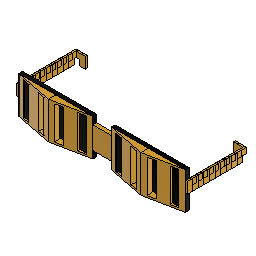
aizawaglasses v3 (Autodesk Fusion 360 design; units mm, degrees)
Autodesk Fusion 360 part; units mm, degrees
sketch "Sketch1" plane through (0, 0, 0) normal (0, 1, 0) x (1, 0, 0) in component "black"
  line L0 (0, 0) -> (50.8, 0)
  line L1 (50.8, 0) -> (50.8, -25.4)
  line L2 (50.8, -25.4) -> (0, -25.4)
  line L3 (0, -25.4) -> (0, 0)
  dimension "d1" = 50.8
  dimension "d2" = 25.4
  constraint horizontal L0
  constraint vertical L1
  constraint horizontal L2
  constraint vertical L3
  constraint coincident L0.start L3.end
  measures "d1" distance of L1.end L2.end
  measures "d2" distance of L0.start L2.end
extrude "Extrude1" add sketch "Sketch1" along normal blind 2.54 makes body 1 in component "black"
sketch "Sketch1 (2)" plane through (0, 0, 0) normal (0, 0, -1) x (1, 0, 0) in component "goggle"
  line L0 (50.8, 0) -> (0, 0)
  line L1 (0, 0) -> (0, -2.54)
  line L2 (0, -2.54) -> (50.8, -2.54)
  line L3 (50.8, -2.54) -> (50.8, 0)
  line L4 (25.4, 0) -> (25.4, 5.08)
  line L5 (25.4, 5.08) -> (50.8, 0)
  dimension "d5" = 5.08
  constraint midpoint L0 L4.start
  constraint perpendicular L0 L4
  constraint coincident L0.start L3.end
  measures "d5" distance of L4.start L4.end
extrude "Extrude1'" add sketch "Sketch1 (2)" against normal blind 25.4 separate body contours L0 L4 L5 makes body 2 in component "goggle"
copy_body "CopyPasteBodies1" bodies 2 makes body 3 in component "goggle"
move_body "Move1" bodies 3 to x (-1, 0, 0) y (0, 1, 0) z (0, 0, -1) at (50.8, 0, 27.056) in component "goggle"
move_body "Move2" bodies 3 to x (1, 0, 0) y (0, 1, 0) z (0, 0, 1) at (0, 0, -1.656) in component "goggle"
sketch "Sketch2" plane through (0, 0, 0) normal (-0.196116, -0.980581, 0) x (0.980581, -0.196116, 0) in component "goggle"
  line L0 (25.903, 25.4) -> (0, 25.4)
  line L1 (0, 25.4) -> (0, 0)
  line L2 (0, 0) -> (25.903, 0)
  line L3 (25.903, 0) -> (25.903, 25.4)
  line L4 (3.81, 24.13) -> (8.89, 24.13)
  line L5 (8.89, 24.13) -> (8.89, 1.27)
  line L6 (8.89, 1.27) -> (3.81, 1.27)
  line L7 (3.81, 1.27) -> (3.81, 24.13)
  line L8 (17.013, 24.13) -> (22.093, 24.13)
  line L9 (22.093, 24.13) -> (22.093, 1.27)
  line L10 (22.093, 1.27) -> (17.013, 1.27)
  line L11 (17.013, 1.27) -> (17.013, 24.13)
  dimension "d8" = 22.86
  dimension "d9" = 5.08
  dimension "d10" = 22.86
  dimension "d11" = 5.08
  dimension "d12" = 3.81
  dimension "d13" = 3.81
  dimension "d14" = 1.27
  dimension "d15" = 1.27
  constraint horizontal L4
  constraint vertical L5
  constraint horizontal L6
  constraint vertical L7
  constraint horizontal L8
  constraint vertical L9
  constraint horizontal L10
  constraint vertical L11
  measures "d8" distance of L8.start L10.end
  measures "d9" distance of L8.start L8.end
  measures "d10" distance of L4.start L6.end
  measures "d11" distance of L4.start L4.end
  measures "d12" distance of L1 L7
  measures "d13" distance of L3 L9
  measures "d14" distance of L0 L4
  measures "d15" distance of L0 L8
extrude "Extrude2" cut sketch "Sketch2" against normal blind 7.62 contours L4 L5 L6 L7 | L8 L9 L10 L11 bodies 3 in component "goggle"
sketch "Sketch3" plane through (1.9538, -9.7692, 0) normal (0.196116, -0.980581, 0) x (0.980581, 0.196116, 0) in component "goggle"
  line L0 (23.9105, 0) -> (49.8135, 0)
  line L1 (49.8135, 0) -> (49.8135, 25.4)
  line L2 (49.8135, 25.4) -> (23.9105, 25.4)
  line L3 (23.9105, 25.4) -> (23.9105, 0)
  line L4 (27.7205, 24.13) -> (32.8005, 24.13)
  line L5 (32.8005, 24.13) -> (32.8005, 1.27)
  line L6 (32.8005, 1.27) -> (27.7205, 1.27)
  line L7 (27.7205, 1.27) -> (27.7205, 24.13)
  line L8 (40.9235, 24.13) -> (46.0035, 24.13)
  line L9 (46.0035, 24.13) -> (46.0035, 1.27)
  line L10 (46.0035, 1.27) -> (40.9235, 1.27)
  line L11 (40.9235, 1.27) -> (40.9235, 24.13)
  dimension "d18" = 22.86
  dimension "d19" = 5.08
  dimension "d20" = 3.81
  dimension "d21" = 1.27
  dimension "d22" = 22.86
  dimension "d23" = 5.08
  dimension "d24" = 1.27
  dimension "d25" = 3.81
  constraint horizontal L4
  constraint vertical L5
  constraint horizontal L6
  constraint vertical L7
  constraint horizontal L8
  constraint vertical L9
  constraint horizontal L10
  constraint vertical L11
  measures "d18" distance of L4.start L6.end
  measures "d19" distance of L4.start L4.end
  measures "d20" distance of L3 L7
  measures "d21" distance of L2 L4
  measures "d22" distance of L8.start L10.end
  measures "d23" distance of L8.start L8.end
  measures "d24" distance of L2 L8
  measures "d25" distance of L1 L9
extrude "Extrude3" cut sketch "Sketch3" against normal blind 10.16 contours L4 L5 L6 L7 | L8 L9 L10 L11 bodies 2 in component "goggle"
sketch "Sketch1 (3)" plane through (50.8, 0, 0) normal (1, 0, 0) x (0, 1, 0)
  line L0 (0, 25.4) -> (0, 0)
  line L1 (0, 0) -> (2.54, 0)
  line L2 (2.54, 0) -> (2.54, 25.4)
  line L3 (2.54, 25.4) -> (0, 25.4)
  line L4 (0, 20.32) -> (2.54, 20.32)
  line L5 (2.54, 20.32) -> (2.54, 5.08)
  line L6 (2.54, 5.08) -> (0, 5.08)
  line L7 (0, 5.08) -> (0, 20.32)
  constraint horizontal L4
  constraint vertical L5
  constraint horizontal L6
  constraint vertical L7
  constraint coincident L2 L5.end
  constraint coincident L0 L4.start
extrude "Extrude1''" add sketch "Sketch1 (3)" along normal blind 12.7 separate body contours L0 L2 L4 L5 L6 L7 makes body 4
copy_body "CutPasteBodies1" bodies 4 removing the originals makes body 5 in component "strap"
copy_body "CopyPasteBodies1'" bodies 2 1 3 makes body 6 makes body 7 makes body 8
move_body "Move1'" bodies 6 7 8 to x (1, 0, 0) y (0, 1, 0) z (0, 0, 1) at (63.5, 0, 0)
sketch "Sketch2 (2)" plane through (114.3, 0, 0) normal (1, 0, 0) x (0, 1, 0) in component "strap"
  line L0 (0, 25.4) -> (0, 0)
  line L1 (0, 0) -> (2.54, 0)
  line L2 (2.54, 0) -> (2.54, 25.4)
  line L3 (2.54, 25.4) -> (0, 25.4)
  line L4 (0, 19.1041) -> (52.113, 19.1041)
  line L5 (52.113, 19.1041) -> (52.113, 11.4841)
  line L6 (52.113, 11.4841) -> (0, 11.4841)
  line L7 (0, 11.4841) -> (0, 19.1041)
  dimension "d30" = 7.62
  constraint horizontal L4
  constraint vertical L5
  constraint horizontal L6
  constraint vertical L7
  constraint coincident L0 L4.start
  measures "d30" distance of L4.start L6.end
sketch "Sketch3 (2)" plane through (114.3, 0, 0) normal (1, 0, 0) x (0, 1, 0) in component "strap"
  line L0 (0, 19.05) -> (3.81, 19.05)
  line L1 (3.81, 19.05) -> (3.81, 11.43)
  line L2 (3.81, 11.43) -> (0, 11.43)
  line L3 (0, 11.43) -> (0, 19.05)
  line L4 (0, 19.05) -> (6.35, 19.05)
  line L5 (6.35, 19.05) -> (6.35, 15.24)
  line L6 (6.35, 15.24) -> (0, 15.24)
  line L7 (0, 15.24) -> (0, 19.05)
  constraint horizontal L0
  constraint vertical L1
  constraint horizontal L2
  constraint vertical L3
  constraint horizontal L4
  constraint vertical L5
  constraint horizontal L6
  constraint vertical L7
extrude "Extrude2'" add sketch "Sketch3 (2)" sketch "Sketch2 (2)" along normal blind 1.27 separate body of sketch 2 contours L0 L2 L4 L6 L7 makes body 9 in component "strap"
copy_body "CutPasteBodies2" bodies 9 removing the originals makes body 10 in component "strap"
sketch "Sketch4" plane through (114.3, 0, 0) normal (1, 0, 0) x (0, 1, 0)
  line L0 (0, 25.4) -> (0, 0)
  line L1 (0, 0) -> (2.54, 0)
  line L2 (2.54, 0) -> (2.54, 25.4)
  line L3 (2.54, 25.4) -> (0, 25.4)
  line L4 (0, 15.24) -> (34.9541, 15.24)
  constraint coincident L0 L4.start
  constraint perpendicular L2 L4
pattern_path "PathPattern1" count 10 spacing 3.8126 from (114.3, 0, 15.24) path "Sketch4" along L4 of bodies 10 makes body 11 at (114.3, 5.0826, 15.258) makes body 12 at (114.7233, 7.6253, 13.988) makes body 13 at (114.7233, 11.4379, 13.988) makes body 14 at (114.7233, 15.2505, 13.988) makes body 15 at (114.7233, 19.0632, 13.988) makes body 16 at (114.7233, 22.8758, 13.988) makes body 17 at (114.7233, 26.6884, 13.988) makes body 18 at (114.7233, 30.5011, 13.988) makes body 19 at (114.7233, 34.3137, 13.988) in component "strap"
copy_body "CopyPasteBodies3" bodies 10 11 12 14 13 15 16 17 18 19 makes body 20 makes body 21 makes body 22 makes body 23 makes body 24 makes body 25 makes body 26 makes body 27 makes body 28 makes body 29 in component "strap"
move_body "Move1''" bodies 20 21 22 23 24 25 26 27 28 29 to x (1, 0, 0) y (0, 1, 0) z (0, 0, 1) at (-116.84, 0, 0) in component "strap"
move_body "Move2'" bodies 26 27 20 23 29 21 28 22 25 24 to x (1, 0, 0) y (0, 1, 0) z (0, 0, 1) at (1.27, 0, 0) in component "strap"
sketch "Sketch5" plane through (0, 40.6654, 0) normal (0, 1, 0) x (-1, 0, 0)
  line L0 (-114.3, 15.24) -> (-114.3, 19.05)
  line L1 (-114.3, 19.05) -> (-115.57, 19.05)
  line L2 (-115.57, 19.05) -> (-115.57, 15.24)
  line L3 (-115.57, 15.24) -> (-114.3, 15.24)
copy_body "CopyPasteBodies2" bodies 19 makes body 30
move_body "Move2''" bodies 30 to x (0, -1, 0) y (1, 0, 0) z (0, 0, 1) at (73.6346, 151.1554, 1.27)
move_body "Move3" bodies 30 to x (1, 0, 0) y (0, 1, 0) z (0, 0, 1) at (0, 5.08, 0)
move_body "Move4" bodies 30 to x (1, 0, 0) y (0, 1, 0) z (0, 0, 1) at (1.27, 0, -1.27)
copy_body "CopyPasteBodies3'" bodies 30 makes body 31
move_body "Move5" bodies 31 to x (1, 0, 0) y (0, 1, 0) z (0, 0, 1) at (-109.22, -1.27, -0.0541)
move_body "Move6" bodies 31 to x (-1, 0, 0) y (0, -1, 0) z (0, 0, 1) at (6.35, 80.0608, 0)
sketch "Sketch6" plane through (0, 39.3954, 0) normal (0, -1, 0) x (1, 0, 0)
  line L0 (6.35, 11.3759) -> (6.35, 19.05)
  line L1 (6.35, 19.05) -> (3.81, 19.05)
  line L2 (3.81, 19.05) -> (3.81, 18.9959)
  line L3 (3.81, 18.9959) -> (0, 18.9959)
  line L4 (0, 18.9959) -> (0, 15.1859)
  line L5 (0, 15.1859) -> (2.54, 15.1859)
  line L6 (2.54, 15.1859) -> (2.54, 11.3759)
  line L7 (2.54, 11.3759) -> (6.35, 11.3759)
  line L8 (0, 22.2006) -> (115.7547, 22.2006)
  constraint perpendicular L4 L8
move_body "Move7" bodies 30 to x (1, 0, 0) y (0, 1, 0) z (0, 0, 1) at (-1.27, -1.27, 0)
sketch "Sketch7" plane through (0, 0, 0) normal (0, 0, 1) x (1, 0, 0)
  circle A0 centre (57.3687, 28.9214) radius 53.4004
component "black" placed x (1, 0, 0) y (0, 1, 0) z (0, 0, 1) at (0, 0, 0)
component "goggle" placed x (1, 0, 0) y (0, 1, 0) z (0, 0, 1) at (0, 0, 0)
component "strap" placed x (1, 0, 0) y (0, 1, 0) z (0, 0, 1) at (0, 0, 0)
